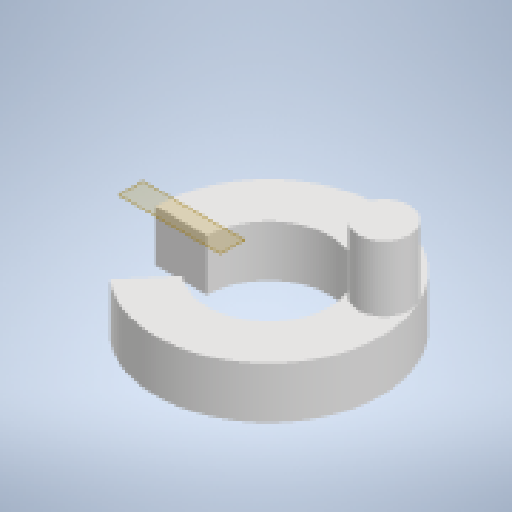
# Autodesk Inventor part: wash_ring
Saved by Autodesk Inventor 2023.3 (Build 273359000, 359)
## iProperties
Created: 2023-11-29
Part Number: wash_ring
Material: Generic
Document SubType Name: Modeling
Designer: mmelin
Density: 1 g/cm^3
Appearance: Default
Author: mmelin
Autodesk Inventor part; units mm, degrees
ref_plane "YZ Plane" through (0, 0, 0) normal (1, 0, 0) x (0, 1, 0)
ref_plane "XZ Plane" through (0, 0, 0) normal (0, 1, 0) x (-1, 0, 0)
ref_plane "XY Plane" through (0, 0, 0) normal (0, 0, 1) x (1, 0, 0)
sketch "Sketch1" plane through (0, 0, 0) normal (0, 0, 1) x (1, 0, 0)
  line L0 (20, 10.9474) -> (20, -17.8312)
  line L1 (-6.604, 6.604) -> (-6.604, -6.604) projected
  line L2 (-6.604, -6.604) -> (6.604, -6.604) projected
  line L3 (6.604, 6.604) -> (-6.604, 6.604) projected
  line L4 (6.604, -6.604) -> (6.604, 6.604) projected
  line L5 (-5.904, -5.904) -> (5.904, -5.904)
  line L6 (5.904, -5.904) -> (5.904, 5.904)
  line L7 (5.904, 5.904) -> (-5.904, 5.904)
  line L8 (-5.904, 5.904) -> (-5.904, -5.904)
  point P0 (0, 0)
  dimension "d2" = 20
  dimension "d8" = 0.7
  dimension "d9" = 0.7
  dimension "d10" = 0.7
  dimension "d11" = 0.7
  constraints: 10 end point, 2 parallel, 1 horizontal, 1 perpendicular, 1 vertical
  measures "d2" distance from line of L0 point (0, 0)
  measures "d8" distance between parallel lines of L1 L8
  measures "d9" distance between parallel lines of L3 L7
  measures "d10" distance between parallel lines of L4 L6
  measures "d11" distance between parallel lines of L2 L5
revolve "Revolution1" add sketch "Sketch1" angle 310 about axis through (20, 10.9474, 0) along (0, -1, 0) contours L8 L7 L6 L5
ref_plane "Work Plane1" through (0, 6.604, 2.5) normal (0, 1, 0) x (0, 0, 1)
sketch "Sketch4" plane through (-5.904, 5.904, 0) normal (0, 1, 0) x (1, 0, 0)
  line L0 (0, 0) -> (11.808, 0) projected
  line L1 (0, 0) -> (51.808, 0) construction
  arc A0 (9.2532, -19.8436) -> (0, 0) centre (25.904, 0) ccw projected
  line L2 (9.2532, -19.8436) -> (42.5548, 19.8436) construction
  line L3 (9.2532, -19.8436) -> (16.8433, -10.7982) construction
  line L4 (11.808, 0) -> (0, 0) construction
  circle A1 centre (43.9932, 8.4352) radius 5.904
  line L5 (43.9932, 8.4352) -> (42.5548, 19.8436)
  line L6 (43.9932, 8.4352) -> (51.808, 0)
  point P0 (5.904, 0)
  dimension "d15" = 11.808
  dimension "d16" = 8.4352
  constraints: 8 end point, 2 collinear, 2 point on circle, 1 centre point, 1 equal length
  measures "d15" diameter of A1
  measures "d16" vertical distance of L5.start L1.end
extrude "Extrusion3" add sketch "Sketch4" along normal blind 15 contours L6 L5 A1 | A1 L5 L6
equation "\"d9\" = d8"
equation "\"d10\" = d8"
equation "\"d11\" = d8"
body "Solid1"
